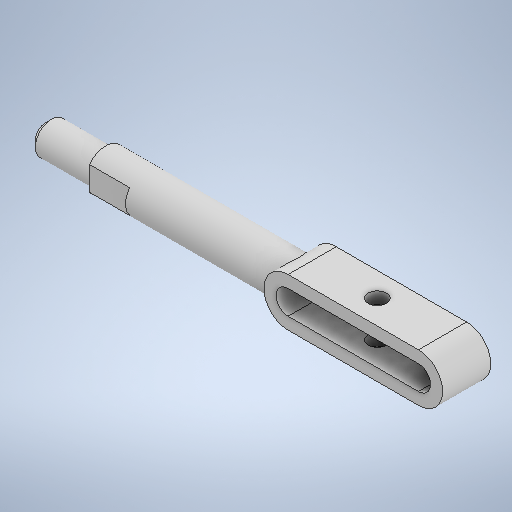
# Autodesk Inventor part: hf2
Saved by Autodesk Inventor 2025 (Build 290162000, 162)
## iProperties
Created: 2025-04-17
Part Number: hf2
Material: Generic
Document SubType Name: Modeling
Designer: Asus
Density: 1 g/cm^3
Appearance: Default
Author: Asus
Autodesk Inventor part; units mm, degrees
sketch "Sketch1" plane through (0, 0, 0) normal (0, 0, 1) x (1, 0, 0)
  line L0 (0, 0) -> (65, 0)
  circle A0 centre (0, 0) radius 12
  circle A1 centre (65, 0) radius 12
  line L1 (0, 12) -> (65, 12)
  line L2 (0, -12) -> (65, -12)
  dimension "d0" = 65
  dimension "d1" = 24
  constraints: 6 end point, 4 point on circle, 3 horizontal, 2 centre point, 2 coincident, 2 tangent, 1 equal radius
  measures "d0" distance of L0.start L0.end
  measures "d1" diameter of A0
extrude "Extrusion1" add sketch "Sketch1" along normal blind 24
sketch "Sketch2" plane through (0, 0, 24) normal (0, 0, 1) x (1, 0, 0)
  circle A0 centre (0, 0) radius 6
  arc A1 (65, -12) -> (65, 12) centre (65, 0) ccw projected
  circle A2 centre (65, 0) radius 6
  line L0 (0, 6) -> (65, 6)
  line L1 (0, -6) -> (65, -6)
  dimension "d4" = 12
  constraints: 4 end point, 4 point on circle, 2 centre point, 2 coincident, 2 horizontal, 2 tangent, 1 equal radius
  measures "d4" diameter of A0
extrude "Extrusion2" cut sketch "Sketch2" against normal through all
sketch "Sketch3" plane through (0, 12, 0) normal (0, 1, 0) x (1, 0, 0)
  point P0 (0, 0)
  point P1 (32.5, -12)
hole "Hole1" at (32.5, 12, 12) direction (0, -1, 0) diameter 9 end through all
ref_plane "Work Plane1" through (-12, 0, 0) normal (1, 0, 0) x (0, 1, 0)
sketch "Sketch4" plane through (-12, 0, 0) normal (1, 0, 0) x (0, 1, 0)
  circle A0 centre (0, 12) radius 10
  point P0 (0, 0)
  dimension "d14" = 20
  constraints: 1 centre point, 1 coincident
  measures "d14" diameter of A0
extrude "Extrusion3" add sketch "Sketch4" along normal blind 6
sketch "Sketch5" plane through (-12, 0, 0) normal (1, 0, 0) x (0, 1, 0)
  arc A0 (0, 22) -> (0, 2) centre (0, 12) ccw projected
  circle A1 centre (0, 12) radius 10
  point P0 (0, 0)
  point P1 (0, 2)
  dimension "d17" = 20
  constraints: 1 centre point, 1 coincident
  measures "d17" diameter of A1
extrude "Extrusion4" add sketch "Sketch5" against normal blind 91
sketch "Sketch6" plane through (-103, 0, 12) normal (-1, 0, 0) x (0, 0, 1)
  circle A0 centre (0, 0) radius 8
  point P0 (-12, 0)
  dimension "d20" = 16
  constraints: 1 centre point
  measures "d20" diameter of A0
extrude "Extrusion5" add sketch "Sketch6" along normal blind 30
chamfer "Chamfer1" distance 3 angle 45 1 edges at (-133, 0, 4) measured on face at (-133, -1.0645, 14.108)
ref_plane "Work Plane2" through (-12, 0, 22) normal (0, 0, 1) x (1, 0, 0)
sketch "Sketch7" plane through (-12, 0, 22) normal (0, 0, 1) x (1, 0, 0)
  line L0 (-91, -10) -> (5.3668, -10) projected
  line L1 (-91, 10) -> (5.3668, 10) projected
  line L2 (-91, 10) -> (-91, -10) projected
  line L3 (-91, -10) -> (-71, -10)
  line L4 (-71, -10) -> (-71, 10)
  line L5 (-71, 10) -> (-91, 10)
  line L6 (-91, 10) -> (-91, -10)
  point P0 (12, 0)
  point P1 (-71, -10)
  dimension "d26" = 20
  constraints: 8 end point, 2 parallel, 1 horizontal, 1 perpendicular, 1 point on line
  measures "d26" distance of L5.end L4.end
extrude "Extrusion6" cut sketch "Sketch7" against normal blind 2
ref_plane "Work Plane3" through (-12, 0, 2) normal (0, 0, 1) x (1, 0, 0)
sketch "Sketch8" plane through (-12, 0, 2) normal (0, 0, 1) x (1, 0, 0)
  line L0 (-91, -10) -> (5.3668, -10) projected
  line L1 (-91, 10) -> (-91, -10) projected
  line L2 (-91, 10) -> (5.3668, 10) projected
  line L3 (-91, -10) -> (-71, -10)
  line L4 (-71, -10) -> (-71, 10)
  line L5 (-71, 10) -> (-91, 10)
  line L6 (-91, 10) -> (-91, -10)
  point P0 (12, 0)
  point P1 (-91, 6)
  point P2 (-91, -6)
  point P3 (-71, -10)
  dimension "d29" = 20
  constraints: 8 end point, 2 parallel, 1 horizontal, 1 perpendicular, 1 point on line
  measures "d29" distance of L5.end L4.end
extrude "Extrusion7" cut sketch "Sketch8" along normal blind 2
body "Solid1"
